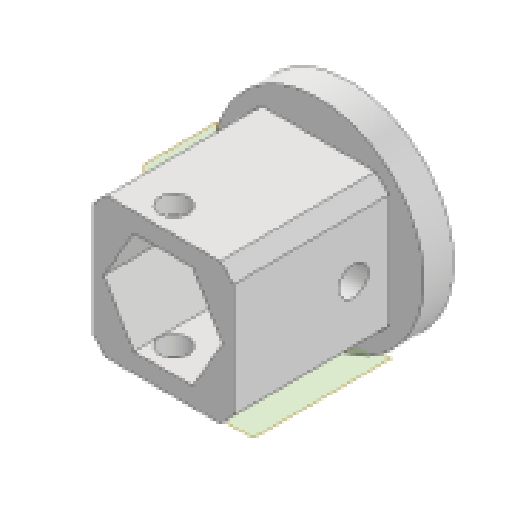
# Autodesk Inventor part: 6mm_shaft_couple_sideclip_v2
Saved by Autodesk Inventor 2023 (Build 270158000, 158)
## iProperties
Created: 2020-09-24
Part Number: 6mm_shaft_couple_sideclip_v2
Material: Generic
Document SubType Name: Modeling
Designer: CDT
Density: 1 g/cm^3
Appearance: Default
Author: CDT
Autodesk Inventor part; units mm, degrees
ref_plane "YZ Plane" through (0, 0, 0) normal (1, 0, 0) x (0, 1, 0)
ref_plane "XZ Plane" through (0, 0, 0) normal (0, 1, 0) x (-1, 0, 0)
ref_plane "XY Plane" through (0, 0, 0) normal (0, 0, 1) x (1, 0, 0)
sketch "Sketch1" plane through (0, 0, 0) normal (0, 0, 1) x (1, 0, 0)
  circle A0 centre (0, 0) radius 9
  line L0 (-0.75, 10) -> (0.75, 10)
  line L1 (0.75, 10) -> (0.75, 0)
  line L2 (0.75, 0) -> (-0.75, 0)
  line L3 (-0.75, 0) -> (-0.75, 10)
  point P0 (-0.75, 8.9687)
  point P1 (0.75, 8.9687)
  dimension "d0" = 18
  dimension "d26" = 0.75
  dimension "d28" = 0
  dimension "d29" = 10
  constraints: 8 end point, 2 parallel, 1 centre point, 1 coincident, 1 horizontal, 1 perpendicular
  measures "d0" diameter of A0
  measures "d26" distance from line of A0.centre L3
  measures "d28" distance from line of point (0, 0) L2
  measures "d29" distance from line of A0.centre L0
extrude "Extrusion1" add sketch "Sketch1" along normal blind 15.5 contours A0 L3 L2 L1 | L1 L2 L3 A0
sketch "Sketch2" plane through (0, 0, 0) normal (0, 0, -1) x (-1, 0, 0)
  line L0 (-1.5, -2.5) -> (1.5, -2.5)
  line L1 (1.5, -2.5) -> (1.5, 2.5)
  line L2 (1.5, 2.5) -> (-1.5, 2.5)
  line L3 (-1.5, 2.5) -> (-1.5, -2.5)
  point P0 (0, 0)
  dimension "d3" = 3
  dimension "d4" = 5
  dimension "d5" = 2.5
  dimension "d6" = 1.5
  constraints: 8 end point, 2 parallel, 1 horizontal, 1 perpendicular
  measures "d3" distance of L2.end L1.end
  measures "d4" distance of L1.end L0.end
  measures "d5" distance from line of L2 point (0, 0)
  measures "d6" distance from line of L3 point (0, 0)
extrude "Extrusion2" cut sketch "Sketch2" against normal blind 10
sketch "Sketch3" plane through (0, 0, 15.5) normal (0, 0, 1) x (1, 0, 0)
  circle A0 centre (0, 0) radius 1.6
  dimension "d9" = 3.2
  constraints: 1 centre point, 1 coincident
  measures "d9" diameter of A0
extrude "Extrusion3" [suppressed]
sketch "Sketch4" plane through (0, 0, 0) normal (0, 0, -1) x (-1, 0, 0)
  circle A0 centre (0, 0) radius 4.5
  dimension "d12" = 9
  constraints: 1 centre point, 1 coincident
  measures "d12" diameter of A0
extrude "Extrusion4" [suppressed]
sketch "Sketch10" plane through (0, 0, 15.5) normal (0, 0, 1) x (1, 0, 0)
  line L0 (2.9589, 5.125) -> (5.9178, 0)
  line L1 (5.9178, 0) -> (2.9589, -5.125)
  line L2 (2.9589, -5.125) -> (-2.9589, -5.125)
  line L3 (-2.9589, -5.125) -> (-5.9178, 0)
  line L4 (-5.9178, 0) -> (-2.9589, 5.125)
  line L5 (-2.9589, 5.125) -> (2.9589, 5.125)
  point P0 (0, 0)
  point P1 (0, 0)
  dimension "d145" = 10.25
  constraints: 12 end point, 1 coincident, 13 other
  measures "d145" distance between parallel lines of L5 L2
extrude "Extrusion7" cut sketch "Sketch10" against normal blind 8.3
ref_plane "Work Plane3" through (0, -9, 0) normal (0, -1, 0) x (1, 0, 0)
sketch "Sketch11" plane through (0, -9, 0) normal (0, -1, 0) x (1, 0, 0)
  circle A0 centre (-1.4401, 13) radius 1.45
  line L0 (9, 15.5) -> (-9, 15.5) projected
  point P0 (0, 0)
  dimension "d66" = 2.9
  dimension "d144" = 2.5
  constraints: 1 centre point
  measures "d66" diameter of A0
  measures "d144" distance from line of L0 A0.centre
extrude "Extrusion8" cut sketch "Sketch11" against normal through all both and the other way through all
ref_plane "Work Plane4" through (-10.5, -2.5, 0) normal (-1, 0, 0) x (0, 0, 1)
sketch "Sketch12" plane through (-10.5, -2.5, 0) normal (-1, 0, 0) x (0, 0, 1)
  circle A0 centre (3.5, 2.5) radius 1.45
  point P0 (0, 2.5)
  dimension "d71" = 2.9
  dimension "d74" = 3.5
  constraints: 1 centre point
  measures "d71" diameter of A0
  measures "d74" distance of point (0, 2.5) A0.centre
extrude "Extrusion9" cut sketch "Sketch12" against normal blind 22
sketch "Sketch13" plane through (0, 0, 0) normal (0, 0, -1) x (-1, 0, 0)
  circle A0 centre (0, 0) radius 9.25
  circle A1 centre (0, 0) radius 4.75
  dimension "d75" = 9.5
  dimension "d78" = 18.5
  constraints: 2 centre point, 2 coincident
  measures "d75" diameter of A1
  measures "d78" diameter of A0
extrude "Extrusion10" [suppressed]
sketch "Sketch14" plane through (0, 0, -3.7) normal (0, 0, -1) x (-1, 0, 0)
  line L0 (-8, -5) -> (-10, -5)
  line L1 (-10, -5) -> (-10, 5)
  line L2 (-10, 5) -> (-8, 5)
  line L3 (-8, 5) -> (-8, -5)
  line L4 (10, -5) -> (8, -5)
  line L5 (8, -5) -> (8, 5)
  line L6 (8, 5) -> (10, 5)
  line L7 (10, 5) -> (10, -5)
  line L8 (8, 8) -> (-8, 8)
  line L9 (-8, 8) -> (-8, 10)
  line L10 (-8, 10) -> (8, 10)
  line L11 (8, 10) -> (8, 8)
  line L12 (8, -10) -> (-5, -10)
  line L13 (-5, -10) -> (-5, -8)
  line L14 (-5, -8) -> (8, -8)
  line L15 (8, -8) -> (8, -10)
  point P0 (0, 0)
  dimension "d79" = 8
  dimension "d80" = 2
  dimension "d81" = 5
  dimension "d82" = 5
  dimension "d83" = 8
  dimension "d84" = 2
  dimension "d85" = 5
  dimension "d86" = 5
  dimension "d89" = 8
  dimension "d90" = 8
  dimension "d91" = 2
  dimension "d92" = 2
  dimension "d93" = 8
  dimension "d94" = 8
  dimension "d95" = 8
  dimension "d96" = 5
  constraints: 32 end point, 8 parallel, 4 horizontal, 4 perpendicular
  measures "d79" distance from line of L5 point (0, 0)
  measures "d80" distance between parallel lines of L7 L5
  measures "d81" distance from line of L4 point (0, 0)
  measures "d82" distance from line of L6 point (0, 0)
  measures "d83" distance from line of L3 point (0, 0)
  measures "d84" distance between parallel lines of L1 L3
  measures "d85" distance from line of L0 point (0, 0)
  measures "d86" distance from line of L2 point (0, 0)
  measures "d89" distance from line of L14 point (0, 0)
  measures "d90" distance from line of L8 point (0, 0)
  measures "d91" distance between parallel lines of L10 L8
  measures "d92" distance between parallel lines of L12 L14
  measures "d93" distance from line of L15 point (0, 0)
  measures "d94" horizontal distance of L10.end point (0, 0)
  measures "d95" distance from line of L9 point (0, 0)
  measures "d96" distance from line of L13 point (0, 0)
extrude "Extrusion11" [suppressed]
sketch "Sketch15" plane through (0, 0, 0) normal (0, 0, -1) x (-1, 0, 0)
  line L0 (10, -10.5) -> (7, -10.5)
  line L1 (7, -10.5) -> (7, 10.5)
  line L2 (7, 10.5) -> (10, 10.5)
  line L3 (10, 10.5) -> (10, -10.5)
  line L4 (-10, -10.5) -> (-7, -10.5)
  line L5 (-7, -10.5) -> (-7, 10.5)
  line L6 (-7, 10.5) -> (-10, 10.5)
  line L7 (-10, 10.5) -> (-10, -10.5)
  line L8 (-9.5, 10.5) -> (9.5, 10.5)
  line L9 (9.5, 10.5) -> (9.5, 7)
  line L10 (9.5, 7) -> (-9.5, 7)
  line L11 (-9.5, 7) -> (-9.5, 10.5)
  line L12 (-1.5, 2.5) -> (1.5, 2.5) projected
  line L13 (-1.5, -2.5) -> (-1.5, 2.5) projected
  line L14 (1.5, 2.5) -> (1.5, -2.5) projected
  line L15 (1.5, -2.5) -> (-1.5, -2.5) projected
  line L16 (-9.5, -7) -> (9.5, -7)
  line L17 (9.5, -7) -> (9.5, -10.5)
  line L18 (9.5, -10.5) -> (-9.5, -10.5)
  line L19 (-9.5, -10.5) -> (-9.5, -7)
  point P0 (0, 0)
  point P1 (-7, 7)
  point P2 (7, 7)
  point P3 (7, -7)
  point P4 (-7, -7)
  dimension "d101" = 8
  dimension "d102" = 8
  dimension "d103" = 8
  dimension "d106" = 8
  dimension "d107" = 8
  dimension "d109" = 8
  dimension "d110" = 8
  dimension "d111" = 8
  dimension "d113" = 8
  dimension "d114" = 8
  dimension "d115" = 3
  dimension "d118" = 7
  dimension "d119" = 7
  dimension "d120" = 7
  dimension "d121" = 7
  dimension "d146" = 3
  constraints: 32 end point, 8 parallel, 4 horizontal, 4 perpendicular
  measures "d101" distance between parallel lines of L11 L13
  measures "d102" distance between parallel lines of L9 L14
  measures "d103" distance between parallel lines of L8 L12
  measures "d106" distance between parallel lines of L2 L12
  measures "d107" distance between parallel lines of L0 L15
  measures "d109" distance between parallel lines of L14 L17
  measures "d110" distance between parallel lines of L15 L18
  measures "d111" distance between parallel lines of L19 L13
  measures "d113" distance between parallel lines of L15 L4
  measures "d114" distance between parallel lines of L6 L12
  measures "d115" distance between parallel lines of L7 L5
  measures "d118" distance from line of L1 point (0, 0)
  measures "d119" distance from line of L10 point (0, 0)
  measures "d120" distance from line of point (0, 0) L5
  measures "d121" distance from line of L16 point (0, 0)
  measures "d146" distance between parallel lines of L3 L1
extrude "Extrusion12" cut sketch "Sketch15" against normal blind 16.25 contours L0 L17 L16 L1 L10 L9 L2 L3 | L0 L1 L16 L17 | L18 L5 L16 L1 | L9 L10 L1 L2 | L4 L19 L16 L5 | L1 L10 L5 L8 | L16 L19 L4 L7 L6 L11 L10 L5 | L5 L10 L11 L6
sketch "Sketch17" plane through (0, 0, 0) normal (0, 0, -1) x (-1, 0, 0)
  line L0 (4.5, 4.5) -> (7, 4.5)
  line L1 (7, 4.5) -> (7, 7)
  line L2 (7, 7) -> (4.5, 7)
  line L3 (4.5, 7) -> (4.5, 4.5)
  line L4 (5.6569, 7) -> (-5.6569, 7) projected
  line L5 (7, -5.6569) -> (7, 5.6569) projected
  line L6 (7, -7) -> (4.5, -7)
  line L7 (4.5, -7) -> (4.5, -4.5)
  line L8 (4.5, -4.5) -> (7, -4.5)
  line L9 (7, -4.5) -> (7, -7)
  line L10 (-7, -7) -> (-4.5, -7)
  line L11 (-4.5, -7) -> (-4.5, -4.5)
  line L12 (-4.5, -4.5) -> (-7, -4.5)
  line L13 (-7, -4.5) -> (-7, -7)
  line L14 (-4.5, 7) -> (-7, 7)
  line L15 (-7, 7) -> (-7, 4.5)
  line L16 (-7, 4.5) -> (-4.5, 4.5)
  line L17 (-4.5, 4.5) -> (-4.5, 7)
  line L18 (-5.6569, -7) -> (5.6569, -7) projected
  line L19 (-7, 5.6569) -> (-7, -5.6569) projected
  point P0 (0, 0)
  point P1 (7, -4.5)
  point P2 (-4.5, 7)
  dimension "d128" = 2.5
  dimension "d129" = 2.5
  dimension "d130" = 2.5
  dimension "d131" = 2.5
  dimension "d132" = 2.5
  dimension "d133" = 2.5
  dimension "d134" = 2.5
  dimension "d135" = 2.5
  constraints: 32 end point, 8 collinear, 8 parallel, 4 horizontal, 4 perpendicular
  measures "d128" distance between parallel lines of L0 L2
  measures "d129" distance between parallel lines of L3 L1
  measures "d130" distance of L7.end L8.end
  measures "d131" distance of L6.end L7.end
  measures "d132" distance of L12.end L11.end
  measures "d133" distance of L11.end L10.end
  measures "d134" distance of L16.end L15.end
  measures "d135" distance of L15.end L14.end
extrude "Extrusion14" [suppressed]
sketch "Sketch18" plane through (0, 0, 0) normal (0, 0, -1) x (-1, 0, 0)
  circle A0 centre (0, 0) radius 10.5
  line L0 (-1.5, -2.5) -> (-1.5, 2.5) projected
  line L1 (1.5, 2.5) -> (1.5, -2.5) projected
  line L2 (-1.5, 2.5) -> (1.5, 2.5)
  line L3 (1.5, 2.5) -> (1.5, -2.5)
  line L4 (1.5, -2.5) -> (-1.5, -2.5)
  line L5 (-1.5, -2.5) -> (-1.5, 2.5)
  dimension "d138" = 21
  constraints: 8 end point, 2 parallel, 1 centre point, 1 coincident, 1 horizontal, 1 perpendicular
  measures "d138" diameter of A0
extrude "Extrusion15" add sketch "Sketch18" along normal blind 3
chamfer "Chamfer1" distance 5 angle 45 4 edges at (-1.5, 0, -3) (1.5, 0, -3) (0, 2.5, -3) (0, -2.5, -3)
equation "\"d5\" = 0.5 * d4"
equation "\"d6\" = 0.5 * d3"
equation "\"d79\" = d83"
equation "\"d84\" = d80"
equation "\"d89\" = d79"
equation "\"d90\" = d79"
equation "\"d91\" = d80"
equation "\"d92\" = d80"
equation "\"d119\" = d118"
equation "\"d120\" = d118"
equation "\"d121\" = d118"
equation "\"d128\" = d129"
equation "\"d130\" = d129"
equation "\"d131\" = d129"
equation "\"d132\" = d129"
equation "\"d133\" = d129"
equation "\"d134\" = d129"
equation "\"d135\" = d129"
body "Solid1"
